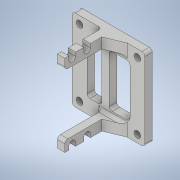
# Autodesk Inventor part: tarto
Saved by Autodesk Inventor 2020 (Build 240168000, 168)
## iProperties
Created: 2019-06-30
Part Number: tarto
Material: Generic
Document SubType Name: Modeling
Designer: Horváth Patrik
Density: 1 g/cm^3
Appearance: Default
Author: Horváth Patrik
Autodesk Inventor part; units mm, degrees
ref_plane "YZ Plane" through (0, 0, 0) normal (1, 0, 0) x (0, 1, 0)
sketch "Sketch1" plane through (0, 0, 0) normal (1, 0, 0) x (0, 1, 0)
  line L0 (0, 0) -> (55, 0)
  line L1 (55, 0) -> (55, 35)
  line L2 (0, 35) -> (0, 0)
  line L3 (7, 35) -> (7, 5)
  line L4 (7, 5) -> (48, 5)
  line L5 (48, 5) -> (48, 35)
  line L6 (55, 35) -> (48, 35)
  line L7 (7, 35) -> (0, 35)
  line L8 (27.5, 5) -> (27.5, 0) construction
  arc A0 (52.5, 32.25) -> (52.5, 27.75) centre (52.5, 30) ccw
  line L9 (52.5, 27.75) -> (55, 27.75)
  line L10 (55, 27.75) -> (55, 32.25)
  line L11 (55, 32.25) -> (52.5, 32.25)
  arc A1 (2.5, 27.75) -> (2.5, 32.25) centre (2.5, 30) ccw
  line L12 (2.5, 27.75) -> (0, 27.75)
  line L13 (0, 32.25) -> (2.5, 32.25)
  arc A2 (52.5, 22.25) -> (52.5, 17.75) centre (52.5, 20) ccw
  line L14 (55, 22.25) -> (52.5, 22.25)
  line L15 (52.5, 17.75) -> (55, 17.75)
  arc A3 (2.5, 17.75) -> (2.5, 22.25) centre (2.5, 20) ccw
  line L16 (2.5, 17.75) -> (0, 17.75)
  line L17 (0, 22.25) -> (2.5, 22.25)
  line L18 (55, 17.75) -> (55, 22.25)
  line L19 (0, 17.75) -> (0, 22.25)
  line L20 (0, 27.75) -> (0, 32.25)
  dimension "d10" = 7
  dimension "d17" = 5
  dimension "d18" = 30
  dimension "d19" = 41
  dimension "d20" = 2.25
  dimension "d21" = 5
  dimension "d22" = 2.5
  dimension "d30" = 10
  constraints: 42 end point, 8 point on circle, 6 parallel, 5 collinear, 5 symmetric about line, 4 centre point, 3 perpendicular, 2 horizontal, 2 midpoint, 2 tangent, 1 point on line, 1 vertical, 17 other
  measures "d10" distance of L1.end L5.end
  measures "d17" distance between parallel lines of L0 L4
  measures "d18" distance between parallel lines of L7 L4
  measures "d19" distance between parallel lines of L3 L5
  measures "d20" radius of A0
  measures "d21" distance from line of L6 A0.centre
  measures "d22" distance of L9.start L9.end
  measures "d30" distance of L9.start L15.start
extrude "Extrusion1" add sketch "Sketch1" along normal blind 5 contours L2 L16 A3 L17 L12 A1 L13 L7 L3 L4 L5 L6 L1 L11 A0 L9 L14 A2 L15 L0
ref_plane "Work Plane4" through (0, 2, 0) normal (0, 0, -1) x (-1, 0, 0)
sketch "Sketch2" plane through (0, 2, 0) normal (0, 0, -1) x (-1, 0, 0)
  line L0 (-5, -2) -> (-5, 53) construction
  line L1 (0, -2) -> (0, 53) construction
  line L2 (20, 53) -> (-29, 53)
  line L3 (-29, 53) -> (-29, -2)
  line L4 (-29, -2) -> (20, -2)
  circle A0 centre (15, 48) radius 2.25
  circle A1 centre (15, 3) radius 2.25
  circle A2 centre (-24, 48) radius 2.25
  circle A3 centre (-24, 3) radius 2.25
  line L5 (0, 25.5) -> (-5, 25.5) construction
  line L6 (0, 53) -> (-5, 53) projected
  line L7 (0, -2) -> (-5, -2) projected
  line L8 (0, 53) -> (-5, 53) projected
  line L9 (20, 43) -> (0, 43)
  line L10 (0, 43) -> (0, 8)
  line L11 (0, 8) -> (20, 8)
  line L12 (-5, 46) -> (-5, 5) projected
  line L13 (-5, 43) -> (-19, 43)
  line L14 (-19, 43) -> (-19, 8)
  line L15 (-19, 8) -> (-5, 8)
  line L16 (-5, 8) -> (-5, 43)
  line L17 (20, -2) -> (20, 8)
  line L18 (20, 43) -> (20, 53)
  line L19 (20, 8) -> (10, 8)
  line L20 (10, 8) -> (10, 43)
  line L21 (10, 43) -> (20, 43)
  line L22 (20, 43) -> (20, 8)
  dimension "d37" = 39
  dimension "d38" = 4.5
  dimension "d40" = 5
  dimension "d41" = 5
  dimension "d42" = 5
  dimension "d58" = 5
  dimension "d59" = 5
  dimension "d60" = 10
  dimension "d61" = 5
  dimension "d62" = 20
  dimension "d63" = 10
  constraints: 34 end point, 8 parallel, 4 centre point, 4 horizontal, 4 perpendicular, 3 collinear, 3 equal radius, 3 point on line, 2 horizontal alignment, 2 midpoint, 2 vertical alignment, 1 other
  measures "d37" distance of A3.centre A1.centre
  measures "d38" diameter of A1
  measures "d40" distance from line of L3 A2.centre
  measures "d41" distance from line of L2 A2.centre
  measures "d42" distance from line of L4 A3.centre
  measures "d58" distance from line of A0.centre L9
  measures "d59" distance from line of A1.centre L11
  measures "d60" distance between parallel lines of L3 L14
  measures "d61" distance from line of L18 A0.centre
  measures "d62" distance between parallel lines of L1 L18
  measures "d63" distance between parallel lines of L22 L20
extrude "Extrusion2" add sketch "Sketch2" against normal blind 5 contours L18 L9 L10 L11 L17 L4 L3 L2 | L22 L11 L20 L9
ref_plane "Work Plane5" through (0, 2, 5) normal (0, 0, 1) x (1, 0, 0)
fillet "Fillet5" radius 2 12 edges at (-10, 10, 2.5) (0, 10, 2.5) (-10, 45, 2.5) (0, 45, 2.5) (5, 45, 2.5) (19, 45, 2.5) (19, 10, 2.5) (-20, 0, 2.5) (-20, 55, 2.5) (29, 0, 2.5) (29, 55, 2.5) (5, 10, 2.5)
chamfer "Chamfer2" distance 12 distance2 5 1 edges at (5, 3.5, 5) measured on face at (5.5, 3.5, 5)
chamfer "Chamfer3" distance 12 distance2 5 1 edges at (5, 51.5, 5) measured on face at (5.5, 51.5, 5)
fillet "Fillet6" radius 2 8 edges at (0, 3.5, 5) (0, 51.5, 5) (2.5, 7, 35) (2.5, 48, 35) (11, 48, 5) (2.5, 48, 5) (11, 7, 5) (2.5, 7, 5)
body "Solid1"
